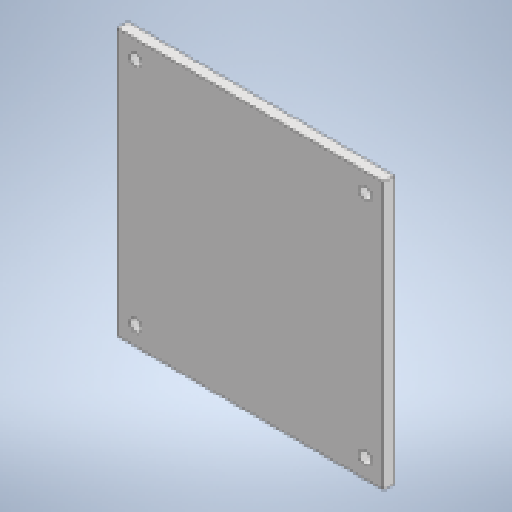
# Autodesk Inventor part: Tapa dispensador
Saved by Autodesk Inventor 2024 (Build 280153000, 153)
## iProperties
Created: 2025-03-02
Part Number: Tapa dispensador
Material: Genérico
Document SubType Name: Modeling
Designer: sergi
Density: 1 g/cm^3
Appearance: Valor por defecto
Author: sergi
Autodesk Inventor part; units mm, degrees
ref_plane "YZ Plane" through (0, 0, 0) normal (1, 0, 0) x (0, 1, 0)
ref_plane "XZ Plane" through (0, 0, 0) normal (0, 1, 0) x (-1, 0, 0)
ref_plane "XY Plane" through (0, 0, 0) normal (0, 0, 1) x (1, 0, 0)
sketch "Boceto1" plane through (0, 0, 0) normal (0, 0, 1) x (1, 0, 0)
  line L0 (-33.5, -15.5) -> (-33.5, 15.5) projected
  line L1 (-36.5, -15.5) -> (-33.5, -15.5) projected
  line L2 (-33.5, 15.5) -> (-36.5, 15.5) projected
  line L3 (-36.5, 15.5) -> (-36.5, -15.5) projected
  line L4 (36.5, -36.5) -> (36.5, 36.5) projected
  line L5 (-36.5, -36.5) -> (36.5, -36.5) projected
  line L6 (-36.5, 36.5) -> (-36.5, -36.5) projected
  line L7 (36.5, 36.5) -> (-36.5, 36.5) projected
  point P0 (0, 0)
extrude "Extrusión1" add sketch "Boceto1" along normal blind 3
sketch "Boceto2" plane through (0, 0, 3) normal (0, 0, 1) x (1, 0, 0)
  line L0 (36.5, 36.5) -> (-36.5, 36.5) projected
  line L1 (-36.5, 36.5) -> (-36.5, -36.5) projected
  line L2 (-36.5, -36.5) -> (36.5, -36.5) projected
  line L3 (36.5, -36.5) -> (36.5, 36.5) projected
  circle A0 centre (-31.4, 31.4) radius 2.1 projected
  circle A1 centre (-31.4, -31.4) radius 2.1 projected
  circle A2 centre (31.4, -31.4) radius 2.1 projected
  circle A3 centre (31.4, 31.4) radius 2.1 projected
  point P0 (0, 0)
hole "Agujero1" at (-31.4, 31.4, 3) at (-31.4, -31.4, 3) at (31.4, -31.4, 3) at (31.4, 31.4, 3) direction (0, 0, -1) diameter 3.2 depth 5
sketch "Boceto4" plane through (-36.5, -36.5, 0) normal (-1, 0, 0) x (0, 0, 1)
  line L0 (0, 73) -> (0, 0) projected
  line L1 (0, 0) -> (3, 0) projected
  line L2 (3, 73) -> (3, 0) projected
  line L3 (0, 73) -> (3, 73) projected
  line L4 (3, 73) -> (0, 73)
  line L5 (0, 73) -> (0, 65)
  line L6 (0, 65) -> (3, 65)
  line L7 (3, 65) -> (3, 73)
  point P0 (0, 36.5)
  dimension "d9" = 8
  constraints: 8 end point, 2 parallel, 1 horizontal, 1 perpendicular, 1 point on line
  measures "d9" distance of L5.end L4.end
extrude "Extrusión2" add sketch "Boceto4" along normal blind 8 contours L3 L2 L6 L0
sketch "Boceto5" plane through (-44.5, -36.5, 0) normal (-1, 0, 0) x (0, 0, 1)
  line L0 (3, 65) -> (3, 73) projected
  line L1 (3, 73) -> (0, 73) projected
  line L2 (0, 73) -> (0, 65) projected
  line L3 (0, 65) -> (3, 65) projected
  line L4 (0, 73) -> (3, 65)
  circle A0 centre (1.5, 69) radius 6
  line L5 (0, 62) -> (3, 62)
  line L6 (3, 62) -> (3, 76)
  line L7 (3, 76) -> (0, 76)
  line L8 (0, 76) -> (0, 62)
  line L9 (0, 62) -> (3, 76) construction
  line L10 (3, 62) -> (0, 76) construction
  point P0 (0, 36.5)
  point P1 (3, 74.8095)
  point P2 (3, 63.1905)
  dimension "d12" = 12
  constraints: 14 end point, 3 midpoint, 2 parallel, 1 centre point, 1 horizontal, 1 perpendicular
  measures "d12" diameter of A0
extrude "Extrusión3" add sketch "Boceto5" along normal blind 3 contours L4 L1 L0 | L6 A0 L8 L3 | L3 L2 L4 | L1 L8 A0 L6 | L8 A0 L2
ref_plane "Plano de trabajo1" through (36.5, 0, 3) normal (0, 1, 0) x (1, 0, 0)
ref_plane "Plano de trabajo2" through (0, -36.5, 0) normal (-1, 0, 0) x (0, 0, 1)
mirror "Simetría1" about plane through (36.5, 0, 3) normal (0, 1, 0) of "Extrusión3", "Extrusión2"
mirror "Simetría2" about plane through (0, -36.5, 0) normal (-1, 0, 0) of "Extrusión3", "Extrusión2", "Simetría1"
sketch "Boceto6" plane through (36.5, -28.5, 0) normal (1, 0, 0) x (0, 0, -1)
  line L0 (0, 13) -> (75, 13) projected
  arc A0 (75, 7) -> (75, 13) centre (75, 10) ccw projected
  line L1 (75, 7) -> (0, 7) projected
  line L2 (0, -8) -> (0, 7) projected
  line L3 (81, -8) -> (0, -8) projected
  line L4 (81, -8) -> (81, 65) projected
  line L5 (81, 65) -> (0, 65) projected
  line L6 (0, 50) -> (0, 65) projected
  line L7 (0, 50) -> (75, 50) projected
  arc A1 (75, 44) -> (75, 50) centre (75, 47) ccw projected
  line L8 (75, 44) -> (0, 44) projected
  line L9 (0, 13) -> (0, 44) projected
  line L10 (0, 44) -> (0, 13) projected
  line L11 (-3, 0) -> (0, 0) projected
  line L12 (0, 0) -> (0, 57) projected
  line L13 (0, 57) -> (-3, 57) projected
  line L14 (-3, 0) -> (-3, 57) projected
  line L15 (3, 35.5) -> (-3, 35.5)
  line L16 (-3, 35.5) -> (-3, 20.5)
  line L17 (-3, 20.5) -> (3, 20.5)
  line L18 (3, 20.5) -> (3, 35.5)
  line L19 (3, 35.5) -> (-3, 20.5) construction
  line L20 (-3, 35.5) -> (3, 20.5) construction
  point P0 (0, 28.5)
  point P1 (0, 28)
  dimension "d15" = 6
  dimension "d16" = 15
  constraints: 12 end point, 2 midpoint, 2 parallel, 1 horizontal, 1 perpendicular
  measures "d15" distance of L17.end L16.end
  measures "d16" distance of L16.end L15.end
extrude "Extrusión4" add sketch "Boceto6" along normal blind 3 contours L17 L14 L15 L9 | L9 L15 L18 L17
mirror "Simetría3" about plane through (0, -36.5, 0) normal (-1, 0, 0) of "Extrusión4"
